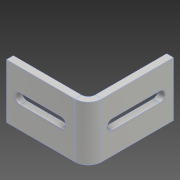
# Autodesk Inventor part: keyL
Saved by Autodesk Inventor 2018 (Build 220112000, 112)
## iProperties
Created: 2018-05-26
Part Number: keyL
Material: アルミニウム 6061
Document SubType Name: Sheet Metal
Designer: NaMACHAN
Mass: 3.45201 g
Surface Area: 16.6707 cm^2
Volume: 1.27852 cm^3
Density: 2.7 g/cm^3
Sheet Metal Rule: AL2mm
Appearance: アルミニウム - フラット
Flat Pattern Width: 1.6 cm
Flat Pattern Length: 4.55239 cm
Flat Pattern Area: 7.28382 cm^2
Sheet Metal Width: 16.000 mm
Sheet Metal Length: 45.524 mm
Sheet Metal Area: 728.382 mm^2
Author: NaMACHAN
Autodesk Inventor part; units mm, degrees
ref_plane "YZ Plane" through (0, 0, 0) normal (1, 0, 0) x (0, 1, 0)
ref_plane "XZ Plane" through (0, 0, 0) normal (0, 1, 0) x (-1, 0, 0)
ref_plane "XY Plane" through (0, 0, 0) normal (0, 0, 1) x (1, 0, 0)
sketch "スケッチ1" plane through (0, 0, 0) normal (0, 1, 0) x (-1, 0, 0)
  line L0 (-10, 8) -> (10, 8)
  line L1 (10, 8) -> (10, -8)
  line L2 (10, -8) -> (-10, -8)
  line L3 (-10, -8) -> (-10, 8)
  line L4 (-10, 8) -> (10, -8) construction
  line L5 (10, 8) -> (-10, -8) construction
  point P0 (0, 0)
  dimension "d0" = 20
  dimension "d1" = 16
  measures "d0" distance of L1.end L2.end
  measures "d1" distance of L0.end L1.end
extrude "プレート1" add sketch "スケッチ1" along normal blind 2
sketch "スケッチ2" plane through (12, 4, -8) normal (1, 0, 0) x (0, 1, 0)
  line L0 (0, 16) -> (0, 0)
  line L1 (0, 0) -> (21, 0)
  line L2 (21, 0) -> (21, 16)
  line L3 (21, 16) -> (0, 16)
  constraints: 6 end point, 1 horizontal, 1 perpendicular, 1 vertical
edge flange "フランジ1" height 25 angle 90 thickness 2 bend radius 2 thickness toward (1, 0, 0) relief tear relief width 2 relief depth 1 edges at (10, 2, 0) wall of the first edge with corners at (12, 4, 8) (12, 4, -8) (12, 25, -8) (12, 25, 8)
bend "曲げ1"
corner "コーナー1"
sketch "スケッチ3" plane through (14, 25, 8) normal (1, 0, 0) x (0, 0, -1)
  line L0 (6.5, -4) -> (6.5, -18)
  arc A0 (6.5, -18) -> (9.5, -18) centre (8, -18) ccw
  line L1 (9.5, -18) -> (9.5, -4)
  arc A1 (9.5, -4) -> (6.5, -4) centre (8, -4) ccw
  line L2 (16, 0) -> (16, -21) projected
  line L3 (0, 0) -> (16, 0) projected
  point P0 (8, -25)
  point P1 (8, 0)
  dimension "d19" = 1.5
  constraints: 4 end point, 4 point on circle, 4 tangent, 2 centre point, 1 midpoint, 1 parallel, 1 vertical, 1 vertical alignment
  measures "d19" radius of A1
extrude "押し出し1" cut sketch "スケッチ3" against normal blind 10
sketch "スケッチ4" plane through (0, 2, 0) normal (0, 1, 0) x (1, 0, 0)
  line L0 (-6, -1.5) -> (6, -1.5)
  arc A0 (6, -1.5) -> (6, 1.5) centre (6, 0) ccw
  line L1 (6, 1.5) -> (-6, 1.5)
  arc A1 (-6, 1.5) -> (-6, -1.5) centre (-6, 0) ccw
  line L2 (-10, -8) -> (-10, 8) projected
  line L3 (10, 8) -> (10, -8) projected
  point P0 (0, 0)
  dimension "d23" = 4
  dimension "d24" = 4
  dimension "d25" = 1.5
  constraints: 4 end point, 4 point on circle, 4 tangent, 2 centre point, 1 horizontal, 1 horizontal alignment, 1 parallel
  measures "d23" distance from line of L2 A1.centre
  measures "d24" distance from line of L3 A0.centre
  measures "d25" radius of A1
extrude "押し出し2" cut sketch "スケッチ4" against normal blind 10
equation "\"d2\" = Thickness"
equation "\"d3\" = BendReliefWidth"
equation "\"d4\" = BendReliefDepth"
equation "\"d5\" = MinimumRemnant"
equation "\"d6\" = TransitionRadius"
equation "\"d9\" = BendRadius"
equation "\"d10\" = CornerReliefSize"
equation "\"d11\" = GapSize"
equation "\"d12\" = JacobiRadiusSize"
equation "\"BendRadius\" = Thickness"
equation "\"BendReliefWidth\" = Thickness"
equation "\"BendReliefDepth\" = 0.5 * Thickness"
equation "\"CornerReliefSize\" = 4 * Thickness"
equation "\"MinimumRemnant\" = 2 * Thickness"
equation "\"TransitionRadius\" = BendRadius"
equation "\"JacobiRadiusSize\" = BendRadius"
equation "\"GapSize\" = Thickness"
equation "\"Thickness\" = 2"
